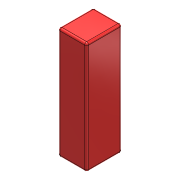
# Autodesk Inventor part: 20_042_BATTERY_R1
Saved by Autodesk Inventor 2021.2 (Build 252289000, 289)
## iProperties
Created: 2018-07-27
Part Number: 20_042_BATTERY_R1
Material: 一般
Document SubType Name: Modeling
Designer: student
Density: 1 g/cm^3
Appearance: 淡い赤
Mass: 104.716 g
Surface Area: 149.636 cm^2
Volume: 104.716 cm^3
Author: student
Autodesk Inventor part; units mm, degrees
ref_plane "YZ Plane" through (0, 0, 0) normal (1, 0, 0) x (0, 1, 0)
ref_plane "XZ Plane" through (0, 0, 0) normal (0, 1, 0) x (-1, 0, 0)
ref_plane "XY Plane" through (0, 0, 0) normal (0, 0, 1) x (1, 0, 0)
sketch "スケッチ1" plane through (0, 0, 0) normal (0, 0, 1) x (1, 0, 0)
  line L0 (-14, 17.25) -> (14, 17.25)
  line L1 (14, 17.25) -> (14, -17.25)
  line L2 (14, -17.25) -> (-14, -17.25)
  line L3 (-14, -17.25) -> (-14, 17.25)
  line L4 (0, 0) -> (0, 17.25) construction
  line L5 (0, 0) -> (14, 0) construction
  dimension "d0" = 28
  dimension "d1" = 34.5
  constraints: 12 end point, 2 horizontal, 2 midpoint, 2 parallel, 1 perpendicular, 1 vertical
  measures "d0" distance of L0.start L0.end
  measures "d1" distance of L0.end L1.end
extrude "押し出し1" add sketch "スケッチ1" along normal mid plane 109
fillet "フィレット1" radius 2 12 edges at (0, 17.25, 54.5) (14, 0, 54.5) (-14, 0, 54.5) (0, -17.25, 54.5) (14, 17.25, 0) (-14, 17.25, 0) (14, -17.25, 0) (14, 0, -54.5) (0, 17.25, -54.5) (-14, -17.25, 0) (-14, 0, -54.5) (0, -17.25, -54.5)
